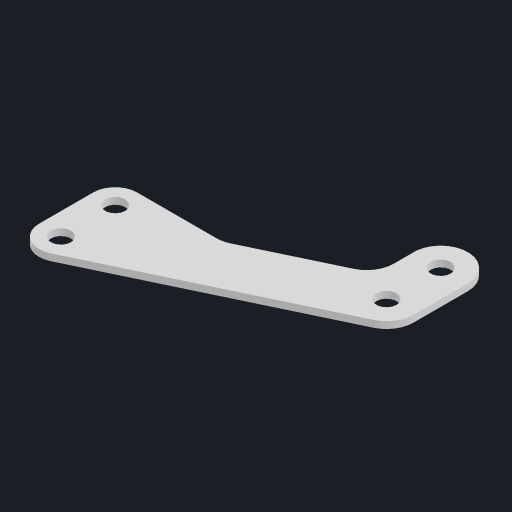
# Autodesk Inventor part: frontgussets
Saved by Autodesk Inventor 2024.2 (Build 282272000, 272)
## iProperties
Created: 2024-01-29
Part Number: frontgussets
Material: Generic
Document SubType Name: Sheet Metal
Designer: reima
Density: 1 g/cm^3
Sheet Metal Rule: Default
Appearance: Default
Author: reima
Autodesk Inventor part; units mm, degrees
ref_plane "YZ Plane" through (0, 0, 0) normal (1, 0, 0) x (0, 1, 0)
ref_plane "XZ Plane" through (0, 0, 0) normal (0, 1, 0) x (-1, 0, 0)
ref_plane "XY Plane" through (0, 0, 0) normal (0, 0, 1) x (1, 0, 0)
sketch "Sketch1" plane through (0, 0, 0) normal (0, 1, 0) x (-1, 0, 0)
  circle A0 centre (15.7792, 0.2535) radius 2.1844 construction
  circle A1 centre (66.5792, 25.6535) radius 2.1844 construction
  circle A2 centre (66.5792, 12.9535) radius 2.1844 construction
  circle A3 centre (15.7792, -12.4465) radius 2.1844 construction
  circle A4 centre (15.7792, -12.4465) radius 2.3495
  circle A5 centre (15.7792, 0.2535) radius 2.3495
  circle A6 centre (66.5792, 12.9535) radius 2.3495
  circle A7 centre (66.5792, 25.6535) radius 2.3495
  line L0 (71.7164, -18.7965) -> (71.7164, 32.0035) construction
  arc A8 (71.7164, 25.6535) -> (64.3805, 30.2964) centre (66.5792, 25.6535) ccw
  arc A9 (9.4292, -12.4465) -> (22.0969, -13.0866) centre (15.7792, -12.4465) ccw
  line L1 (71.7164, 12.9535) -> (71.7164, 25.6535)
  line L2 (9.4292, -12.4465) -> (9.4292, 0.2535)
  line L3 (13.0614, 5.9925) -> (64.3805, 30.2964)
  line L4 (66.5792, 7.8164) -> (48.0123, 7.8164)
  line L5 (25.729, -2.0605) -> (45.2945, 7.2054)
  line L6 (22.0969, -13.0866) -> (22.0969, -7.7995)
  arc A10 (13.0614, 5.9925) -> (9.4292, 0.2535) centre (15.7792, 0.2535) ccw
  arc A11 (66.5792, 7.8164) -> (71.7164, 12.9535) centre (66.5792, 12.9535) ccw
  arc A12 (48.0123, 7.8164) -> (45.2945, 7.2054) centre (48.0123, 1.4664) ccw
  arc A13 (25.729, -2.0605) -> (22.0969, -7.7995) centre (28.4469, -7.7995) ccw
  point P0 (0, 0)
  dimension "d0" = 4.699
  dimension "d1" = 4.699
  dimension "d2" = 4.699
  dimension "d3" = 4.699
  dimension "d5" = 12.7
  dimension "d7" = 6.35
  dimension "d8" = 6.35
  dimension "d9" = 12.7
  measures "d0" diameter of A4
  measures "d1" diameter of A5
  measures "d2" diameter of A6
  measures "d3" diameter of A7
  measures "d5" diameter of A9
  measures "d7" radius of A12
  measures "d8" radius of A10
  measures "d9" distance between parallel lines of L3 L5
extrude "Plate1" add sketch "Sketch1" along normal blind 1.5875
equation "\"d10\" = Thickness"
equation "\"BendRadius\" = Thickness"
equation "\"BendReliefWidth\" = Thickness"
equation "\"BendReliefDepth\" = 0.5 * Thickness"
equation "\"CornerReliefSize\" = 4 * Thickness"
equation "\"MinimumRemnant\" = 2 * Thickness"
equation "\"TransitionRadius\" = BendRadius"
equation "\"JacobiRadiusSize\" = BendRadius"
equation "\"GapSize\" = Thickness"
equation "\"Thickness\" = 1.5875"
body "Solid1"
